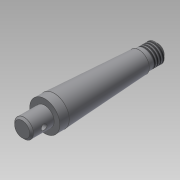
# Autodesk Inventor part: Рукоятка
Saved by Autodesk Inventor 2014 SP1 (Build 180222100, 222)
## iProperties
Created: 2014-04-11
Part Number: Рукоятка
Material: Типовые
Document SubType Name: Modeling
Designer: Украинцев
Mass: 9.12465 g
Surface Area: 31.7802 cm^2
Volume: 9.12465 cm^3
Density: 1 g/cm^3
Appearance: По умолчанию
Author: Украинцев
Autodesk Inventor part; units mm, degrees
ref_plane "YZ Plane" through (0, 0, 0) normal (1, 0, 0) x (0, 1, 0)
ref_plane "XZ Plane" through (0, 0, 0) normal (0, 1, 0) x (-1, 0, 0)
ref_plane "XY Plane" through (0, 0, 0) normal (0, 0, 1) x (1, 0, 0)
sketch "Эскиз1" plane through (0, 0, 0) normal (0, 0, 1) x (1, 0, 0)
  line L0 (0, 0) -> (0, 72)
  line L1 (0, 72) -> (5, 72)
  line L2 (5, 72) -> (5, 62)
  line L3 (5, 62) -> (5.5, 62)
  line L4 (5.5, 62) -> (8, 17)
  line L5 (8, 17) -> (8, 12)
  line L6 (8, 12) -> (5, 12)
  line L7 (5, 12) -> (5, 0)
  line L8 (5, 0) -> (0, 0)
  line L9 (-5, 0) -> (-5, 12) construction
  line L10 (-5, 4) -> (6, 6.9474)
  line L11 (-5, 2.4471) -> (6, 5.3945)
  line L12 (-5, 4) -> (-5, 2.4471)
  line L13 (6, 6.9474) -> (6, 5.3945)
  dimension "d0" = 72
  dimension "d1" = 10
  dimension "d2" = 45
  dimension "d3" = 16
  dimension "d4" = 10
  dimension "d5" = 12
  dimension "d6" = 11
  dimension "d7" = 10
  dimension "d8" = 10
  dimension "d9" = 8
  dimension "d10" = 3
  dimension "d11" = 15
  dimension "d14" = 1
  constraints: 28 end point, 6 parallel, 3 perpendicular, 2 collinear, 2 horizontal alignment, 2 point on line, 1 vertical
  measures "d0" distance of L0.start L0.end
  measures "d1" diameter of L2 L0
  measures "d2" vertical distance of L3.end L4.end
  measures "d3" diameter of L4.end L0
  measures "d4" diameter of L7 L0
  measures "d5" distance of L6.end L7.end
  measures "d6" diameter of L3.end L0
  measures "d7" distance of L1.end L2.end
  measures "d8" diameter of L9 L0
  measures "d9" vertical distance of L10.start L6.end
  measures "d10" diameter of L11 L10
  measures "d11" angle of L8 L10
  measures "d14" distance between parallel lines of L7 L13
revolve "Вращение1" add sketch "Эскиз1" angle 360 about axis through (0, 0, 0) along (0, 1, 0) contours L0 L11 L7 L8 | L0 L10 L7 L11 | L0 L1 L2 L3 L4 L5 L6 L7 L10
revolve "Вращение2" cut sketch "Эскиз1" angle 360 about axis through (-5, 4, 0) along (0.9659258, 0.258819, 0) contours L11 L12 L10 L0 | L0 L10 L7 L11 | L7 L10 L13 L11
thread "Резьба1" size "M10x1.5" class "6g" standard "ANSI Metric M Profile" length 7.5
chamfer "Фаска1" distance 1.6 angle 45 1 edges at (-5, 72, 0)
chamfer "Фаска2" distance 1 angle 45 1 edges at (-5, 0, 0)
equation "\"d8\" = d4"
